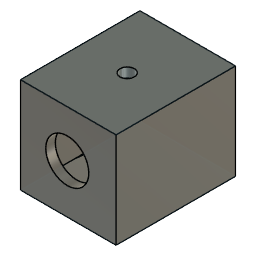
Ewi_Enclosure (Autodesk Fusion 360 archive; units mm, degrees)
design "Moisture Trap 1"
Autodesk Fusion 360 part; units mm, degrees
sketch "Sketch1" plane through (0, 0, 0) normal (0, 0, 1) x (1, 0, 0)
  line L0 (0, 0) -> (20, 0)
  line L1 (20, 0) -> (20, 25)
  line L2 (20, 25) -> (0, 25)
  line L3 (0, 25) -> (0, 0)
  constraint coincident L0.start L3.end
  constraint horizontal L0
  constraint perpendicular L0 L1
  constraint perpendicular L1 L2
  constraint perpendicular L0 L3
extrude "Extrude1" add sketch "Sketch1" along normal blind 20
sketch "Sketch2" plane through (0, 0, 0) normal (0, 0, -1) x (1, 0, 0)
  line L0 (0, 0) -> (0, -25)
  line L1 (0, -25) -> (20, -25)
  line L2 (20, -25) -> (20, 0)
  line L3 (20, 0) -> (0, 0)
shell "Shell1" thickness 2 removed faces 0 bodies 1
sketch "Sketch3" plane through (0, 0, 20) normal (0, 0, 1) x (-1, 0, 0)
  line L0 (0, -25) -> (0, 0)
  line L1 (0, 0) -> (-20, 0)
  line L2 (-20, 0) -> (-20, -25)
  line L3 (-20, -25) -> (0, -25)
hole "Hole1" at (9.9202, 12.4035, 20) direction (0, 0, -1) diameter 3 depth 25 tip angle 118
hole "Hole2" at (9.8027, 0, 10.2267) direction (0, 1, 0) diameter 9 depth 4 tip angle 118
sketch "Sketch4" plane through (20, 0, 0) normal (1, 0, 0) x (0, 1, 0)
  line L0 (0, 0) -> (25, 0)
  line L1 (25, 0) -> (25, 20)
  line L2 (25, 20) -> (0, 20)
  line L3 (0, 20) -> (0, 0)
  line L4 (12.5, 0.7539) -> (2, 2)
  line L5 (2, 2) -> (23, 2)
  line L6 (23, 2) -> (12.5, 0.7539)
  line L7 (2, 2) -> (23, 2)
  line L8 (2, 2) -> (12.5, 0.7539)
  line L9 (23, 2) -> (12.5, 0.7539)
  constraint perpendicular L3 L5
extrude "Extrude2" cut sketch "Sketch4" against normal blind 18 from surface at -1 contours L4 L5 L6 L7 L8 L9
sketch "Sketch5" plane through (0, 25, 0) normal (0, 1, 0) x (-1, 0, 0)
  line L0 (-20, 0) -> (0, 0)
  line L1 (0, 0) -> (0, 20)
  line L2 (0, 20) -> (-20, 20)
  line L3 (-20, 20) -> (-20, 0)
  line L4 (-10, 0.754) -> (-18, 2)
  line L5 (-18, 2) -> (-2, 2)
  line L6 (-2, 2) -> (-10, 0.754)
